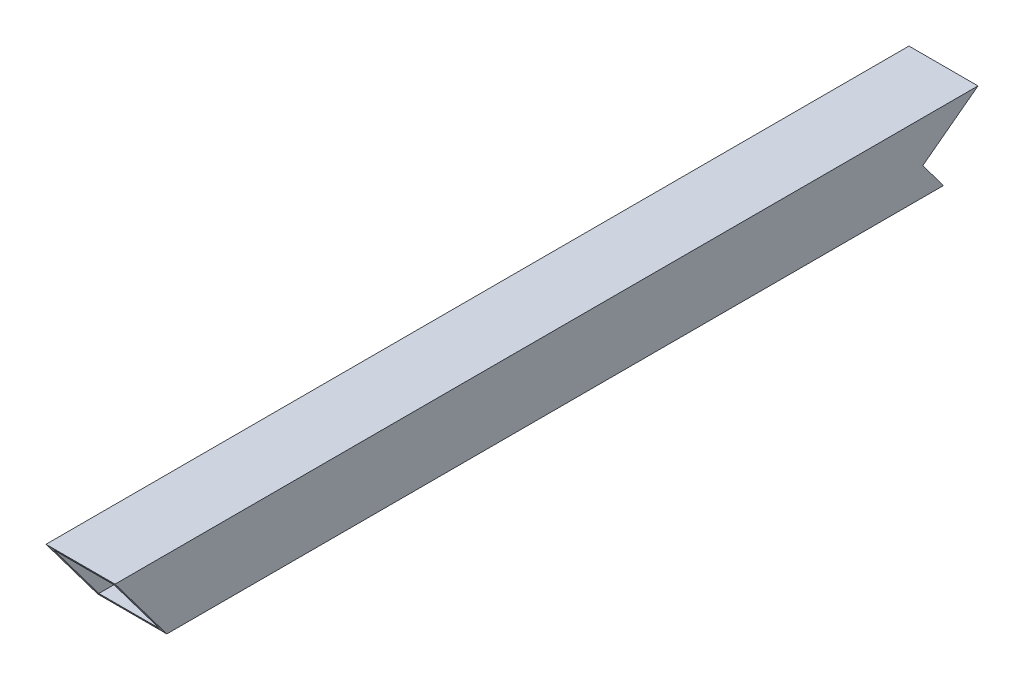
# Autodesk Inventor part: angle support
Saved by Autodesk Inventor 2016 (Build 200138000, 138)
## iProperties
Created: 2016-02-04
Part Number: angle support
Material: Aluminum 6061
Document SubType Name: Modeling
Designer: gus
Density: 2.7 g/cm^3
Appearance: Aluminum - Flat
Author: gus
Autodesk Inventor part; units mm, degrees
ref_plane "YZ Plane" through (0, 0, 0) normal (1, 0, 0) x (0, 1, 0)
ref_plane "XZ Plane" through (0, 0, 0) normal (0, 1, 0) x (-1, 0, 0)
ref_plane "XY Plane" through (0, 0, 0) normal (0, 0, 1) x (1, 0, 0)
sketch "Sketch1" plane through (0, 0, 0) normal (0, 0, 1) x (1, 0, 0)
  line L0 (0, 0) -> (25.4, 0)
  line L1 (25.4, 0) -> (25.4, 25.4)
  line L2 (25.4, 25.4) -> (0, 25.4)
  line L3 (0, 25.4) -> (0, 0)
  line L4 (1.5875, 23.8125) -> (23.8125, 23.8125)
  line L5 (23.8125, 23.8125) -> (23.8125, 1.5875)
  line L6 (23.8125, 1.5875) -> (1.5875, 1.5875)
  line L7 (1.5875, 1.5875) -> (1.5875, 23.8125)
  dimension "d0" = 25.4
  dimension "d1" = 25.4
  dimension "d2" = 1.5875
  constraints: 16 end point, 4 parallel, 2 perpendicular, 1 horizontal, 3 other
  measures "d0" distance of L2.end L1.end
  measures "d1" distance of L1.end L0.end
  measures "d2" distance between parallel lines of L2 L4
extrude "Extrusion1" add sketch "Sketch1" along normal blind 317.5
sketch "Sketch2" plane through (25.4, 0, 0) normal (1, 0, 0) x (0, 0, -1)
  line L0 (0, 0) -> (0, 25.4) projected
  line L1 (0, 25.4) -> (0, 0)
  line L2 (0, 25.4) -> (-317.5, 25.4) projected
  line L3 (-317.5, 25.4) -> (-298.45, 0)
  line L4 (-317.5, 23.8125) -> (-317.5, 1.5875) projected
  line L5 (-298.45, 0) -> (-317.5, 0)
  line L6 (-317.5, 0) -> (-317.5, 25.4) projected
  line L7 (-317.5, 25.4) -> (-317.5, 0)
  line L8 (0, 25.4) -> (-20.32, 10.16)
  line L9 (-20.32, 10.16) -> (-12.7, 0)
  line L10 (0, 0) -> (-317.5, 0) projected
  line L11 (-12.7, 0) -> (0, 0)
  dimension "d6" = 36.87
  dimension "d9" = 53.13
  dimension "d10" = 25.4
  constraints: 14 end point, 3 collinear, 2 point on line, 1 perpendicular
  measures "d6" angle of L4 L3
  measures "d9" angle of L0 L8
  measures "d10" distance of L0.end L8.end
extrude "Extrusion3" cut sketch "Sketch2" against normal blind 25.4 contours L10 L9 L8 L0 | L3 L5 L6 L4
body "Solid1"
